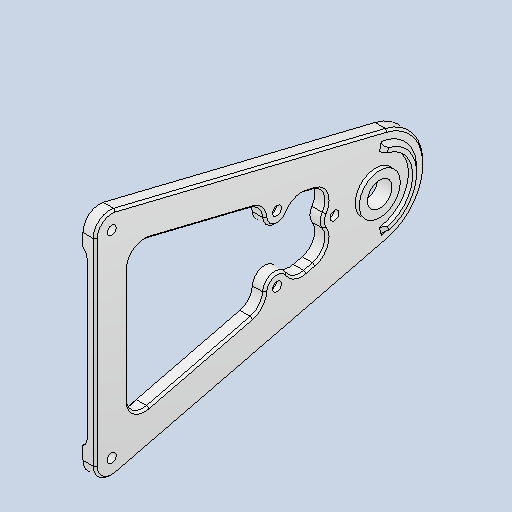
# Autodesk Inventor part: Upright - Blank
Saved by Autodesk Inventor 2023.2 (Build 272271000, 271)
## iProperties
Created: 2023-07-17
Part Number: Upright - Blank
Material: Aluminum 6061
Document SubType Name: Modeling
Designer: Nathan Cai
Mass: 56.1067 g
Surface Area: 124.558 cm^2
Volume: 20.7802 cm^3
Density: 2.7 g/cm^3
Appearance: Aluminum - Flat
Author: Nathan Cai
Autodesk Inventor part; units mm, degrees
ref_plane "YZ Plane" through (0, 0, 0) normal (1, 0, 0) x (0, 1, 0)
ref_plane "XZ Plane" through (0, 0, 0) normal (0, 1, 0) x (-1, 0, 0)
ref_plane "XY Plane" through (0, 0, 0) normal (0, 0, 1) x (1, 0, 0)
sketch "Sketch1" plane through (0, 0, 0) normal (1, 0, 0) x (0, 1, 0)
  circle A0 centre (0, 0) radius 3.5 construction
  circle A1 centre (38.1, -6.35) radius 1.7526
  circle A2 centre (38.1, -6.35) radius 6.35
  line L0 (0, 0) -> (0, -108.2802) construction
  circle A3 centre (0, -108.2802) radius 4.7625
  circle A4 centre (0, -108.2802) radius 19.05
  circle A5 centre (0, -92.4052) radius 1.7526
  circle A6 centre (0, -92.4052) radius 4.7625
  line L1 (44.2669, -7.8639) -> (18.5007, -112.8219)
  line L2 (31.9331, -4.8361) -> (10.4489, -92.3515)
  circle A7 centre (12.7, -70.1802) radius 1.7526
  circle A8 centre (12.7, -70.1802) radius 4.7625
  circle A9 centre (-38.1, -6.35) radius 1.7526
  circle A10 centre (-38.1, -6.35) radius 6.35
  line L3 (-44.2669, -7.8639) -> (-18.5007, -112.8219)
  line L4 (-31.9331, -4.8361) -> (-10.4489, -92.3515)
  circle A11 centre (-12.7, -70.1802) radius 1.7526
  circle A12 centre (-12.7, -70.1802) radius 4.7625
  line L5 (-38.1, 0) -> (38.1, 0)
  line L6 (38.1, -12.7) -> (-38.1, -12.7)
  point P0 (39.9083, -0.2629)
  point P1 (-39.9083, -0.2629)
  point P2 (-18.5007, -112.8219)
  point P3 (16.5723, -67.4078)
  point P4 (14.8483, -74.4306)
  point P5 (3.8683, -89.6271)
  point P6 (-3.8683, -89.6271)
  point P7 (-10.4489, -92.3515)
  point P8 (-14.8483, -74.4306)
  point P9 (-16.5723, -67.4078)
  point P10 (-30.0026, -12.7)
  point P11 (30.0026, -12.7)
  dimension "d0" = 7
  dimension "d2" = 3.5052
  dimension "d3" = 12.7
  dimension "d4" = 38.1
  dimension "d5" = 6.35
  dimension "d6" = 108.2802
  dimension "d7" = 9.525
  dimension "d8" = 38.1
  dimension "d9" = 3.5052
  dimension "d10" = 9.525
  dimension "d11" = 15.875
  dimension "d12" = 12.7
  dimension "d13" = 3.5052
  dimension "d14" = 9.525
  dimension "d15" = 12.7
  dimension "d16" = 38.1
  constraints: 14 end point, 13 centre point, 12 point on circle, 9 coincident, 9 symmetric about line, 6 tangent, 1 parallel, 1 point on line, 1 vertical, 4 other
  measures "d0" diameter of A0
  measures "d2" diameter of A1
  measures "d3" diameter of A2
  measures "d4" horizontal distance of L0.start A1.centre
  measures "d5" vertical distance of L0.start A1.centre
  measures "d6" distance of L0.start L0.end
  measures "d7" diameter of A3
  measures "d8" diameter of A4
  measures "d9" diameter of A5
  measures "d10" diameter of A6
  measures "d11" distance of A3.centre A6.centre
  measures "d12" distance between parallel lines of L1 L2
  measures "d13" diameter of A7
  measures "d14" diameter of A8
  measures "d15" distance from line of L0 A8.centre
  measures "d16" vertical distance of A3.centre A8.centre
extrude "Extrusion1" add sketch "Sketch1" along normal blind 4.7625 contours A2 | A2 L2 L6 L4 A10 L5 | L1 A4 L2 A8 L6 A2 | A2 L6 L2 | A10 | A4 A6 | L4 L6 A10 | A10 L6 L4 A12 A4 L3 | A8 L2 | L2 A8 | A12 L4 | L4 A12 | A6 A4 | A4 A6
fillet "Fillet1" radius 6.35 10 edges at (2.3813, 16.5723, -67.4078) (2.3813, 14.8483, -74.4306) (2.3813, 3.8683, -89.6271) (2.3813, -3.8683, -89.6271) (2.3813, -14.8483, -74.4306) (2.3813, -16.5723, -67.4078) (2.3813, 10.4489, -92.3515) (2.3813, -10.4489, -92.3515) (2.3813, -30.0026, -12.7) (2.3813, 30.0026, -12.7)
sketch "Sketch2" plane through (4.7625, 0, 0) normal (1, 0, 0) x (0, 0, -1)
  circle A0 centre (108.2802, 0) radius 4.7625 projected
  circle A1 centre (108.2802, 0) radius 14.2875
  circle A2 centre (108.2802, 0) radius 12.7
  arc A3 (112.8219, -18.5007) -> (112.8219, 18.5007) centre (108.2802, 0) ccw projected
  line L0 (108.2802, 0) -> (112.8219, -18.5007)
  line L1 (112.8219, 18.5007) -> (7.8639, 44.2669) projected
  line L2 (108.2802, 0) -> (112.8219, 18.5007)
  point P0 (0, 0)
  point P1 (111.6865, 13.8755)
  point P2 (111.308, 12.3338)
  point P3 (111.308, -12.3338)
  point P4 (111.6865, -13.8755)
  point P5 (92.4719, -3.8683)
  point P6 (92.4719, 3.8683)
  dimension "d20" = 28.575
  dimension "d21" = 1.5875
  constraints: 4 end point, 2 centre point, 1 coincident, 1 perpendicular
  measures "d20" diameter of A1
  measures "d21" radial gap between concentric circles of A1 A2
extrude "Extrusion2" add sketch "Sketch2" along normal blind 1.5875 contours L2 A1 L0 A2 picked at (121.358, 4.0209)
fillet "Fillet2" radius 1.5875 1 edges at (4.7625, 0, -122.5677)
chamfer "Chamfer1" distance 1.5875 angle 45 4 edges at (4.7625, -14.6463, -111.8757) (4.7625, -13.1046, -111.4973) (4.7625, 14.6463, -111.8757) (4.7625, 13.1046, -111.4973)
sketch "Sketch3" plane through (0, 0, 0) normal (-1, 0, 0) x (0, 0, 1)
  circle A0 centre (-108.2802, 0) radius 4.7625 projected
  circle A1 centre (-108.2802, 0) radius 11.1125
  arc A2 (-7.8639, -44.2669) -> (0, -38.1) centre (-6.35, -38.1) ccw projected
  line L0 (0, 38.1) -> (0, -38.1) projected
  arc A3 (0, 38.1) -> (-7.8639, 44.2669) centre (-6.35, 38.1) ccw projected
  line L1 (-112.8219, 18.5007) -> (-7.8639, 44.2669) projected
  arc A4 (-112.8219, 18.5007) -> (-112.8219, -18.5007) centre (-108.2802, 0) ccw projected
  line L2 (-7.8639, -44.2669) -> (-112.8219, -18.5007) projected
  circle A5 centre (-6.35, -38.1) radius 1.7526 projected
  circle A6 centre (-92.4052, 0) radius 1.7526 projected
  circle A7 centre (-70.1802, 12.7) radius 1.7526 projected
  arc A8 (-84.6746, 12.3335) -> (-88.4433, 2.6428) centre (-83.1607, 6.1666) ccw projected
  line L3 (-81.2393, 13.1768) -> (-84.6746, 12.3335) projected
  arc A9 (-74.271, 10.2614) -> (-81.2393, 13.1768) centre (-79.7254, 7.0099) ccw projected
  arc A10 (-74.271, 10.2614) -> (-65.4252, 12.433) centre (-70.1802, 12.7) ccw projected
  arc A11 (-60.5991, 18.2438) -> (-65.4252, 12.433) centre (-59.0852, 12.0769) ccw projected
  line L4 (-20.5639, 28.0721) -> (-60.5991, 18.2438) projected
  arc A12 (-12.7, 21.9052) -> (-20.5639, 28.0721) centre (-19.05, 21.9052) ccw projected
  line L5 (-12.7, -21.9052) -> (-12.7, 21.9052) projected
  arc A13 (-20.5639, -28.0721) -> (-12.7, -21.9052) centre (-19.05, -21.9052) ccw projected
  line L6 (-60.5991, -18.2438) -> (-20.5639, -28.0721) projected
  arc A14 (-65.4252, -12.433) -> (-60.5991, -18.2438) centre (-59.0852, -12.0769) ccw projected
  arc A15 (-65.4252, -12.433) -> (-74.271, -10.2614) centre (-70.1802, -12.7) ccw projected
  arc A16 (-81.2393, -13.1768) -> (-74.271, -10.2614) centre (-79.7254, -7.0099) ccw projected
  line L7 (-84.6746, -12.3335) -> (-81.2393, -13.1768) projected
  arc A17 (-88.4433, -2.6428) -> (-84.6746, -12.3335) centre (-83.1607, -6.1666) ccw projected
  arc A18 (-88.4433, -2.6428) -> (-88.4433, 2.6428) centre (-92.4052, 0) ccw projected
  circle A19 centre (-70.1802, -12.7) radius 1.7526 projected
  circle A20 centre (-108.2802, 0) radius 4.7625 projected
  circle A21 centre (-6.35, 38.1) radius 1.7526 projected
  line L8 (-20.5639, 28.0721) -> (0, 33.1203)
  line L9 (0, 38.1) -> (0, -38.1) projected
  line L10 (-20.5639, 28.0721) -> (-60.5991, 18.2438) projected
  line L11 (-92.4052, 0) -> (0, 0) construction
  line L12 (-12.7, -21.9052) -> (-12.7, 21.9052) projected
  line L13 (-20.5639, -28.0721) -> (0, -33.1203)
  point P0 (0, -33.1203)
  point P1 (0, 33.1203)
  dimension "d31" = 22.225
  constraints: 6 end point, 1 centre point, 1 coincident, 1 collinear, 1 perpendicular, 1 point on line, 1 symmetric about line
  measures "d31" diameter of A1
extrude "Extrusion3" cut sketch "Sketch3" against normal blind 0.7937 contours A0 | A1
extrude "Extrusion4" cut sketch "Sketch3" against normal blind 1.5875 contours L13 A13 L5 A12 L8 L0
fillet "Fillet3" radius 3.175 2 edges at (1.5875, 30.5962, -10.282) (1.5875, -30.5962, -10.282)
sketch "Sketch4" plane through (4.7625, 0, 0) normal (1, 0, 0) x (0, 0, -1)
  circle A0 centre (108.2802, 0) radius 4.7625 projected
  circle A1 centre (108.2802, 0) radius 7.9375
  point P0 (0, 0)
  dimension "d38" = 15.875
  constraints: 1 centre point, 1 coincident
  measures "d38" diameter of A1
extrude "Extrusion5" add sketch "Sketch4" along normal blind 1.5875
chamfer "Chamfer2" distance 0.7937 angle 45 22 edges at (4.7625, -31.3838, -60.3429) (4.7625, 0, -127.3302) (4.7625, 31.3838, -60.3429) (4.7625, 43.0968, -2.4315) (4.7625, 0, 0) (4.7625, -43.0968, -2.4315) (4.7625, -12.8679, -77.2745) (4.7625, -12.755, -82.9577) (4.7625, -8.4681, -89.0798) (4.7625, 0, -87.6427) (4.7625, 8.468, -89.0798) (4.7625, 12.755, -82.9577) (4.7625, 12.8679, -77.2745) (4.7625, 8.0748, -69.0448) (4.7625, 16.134, -63.9701) (4.7625, 23.1579, -40.5815) (4.7625, 26.902, -15.1315) (4.7625, 0, -12.7) (4.7625, -26.902, -15.1315) (4.7625, -23.1579, -40.5815) (4.7625, -16.134, -63.9701) (4.7625, -8.0748, -69.0448)
chamfer "Chamfer3" distance 2.54 angle 49 3 edges at (0, -14.4526, -70.1802) (0, 10.9474, -70.1802) (0, -1.7526, -92.4052) measured on face at (0, -2.2526, -92.4052) measured on face at (0, 10.4474, -70.1802) measured on face at (0, -14.9526, -70.1802)
equation "\"d4\" = S_Offset"
equation "\"d5\" = M2S"
equation "\"d6\" = C2C"
equation "\"d7\" = Bore"
equation "\"d8\" = FrontOD"
equation "\"d11\" = Leg_X_Front"
equation "\"d15\" = Leg_Y_Back"
equation "\"d16\" = Leg_X_Back"
equation "\"S_Offset\" = 38.1"
equation "\"M2S\" = 6.35"
equation "\"C2C\" = 108.2802"
equation "\"Bore\" = 9.525"
equation "\"FrontOD\" = 38.1"
equation "\"Leg_X_Front\" = 15.875"
equation "\"Leg_Y_Back\" = 12.7"
equation "\"Leg_X_Back\" = 38.1"
body "Solid1"
